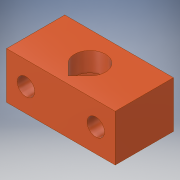
# Autodesk Inventor part: X-axis Holder coupler
Saved by Autodesk Inventor 2018 (Build 220112000, 112)
## iProperties
Created: 2013-10-26
Part Number: X-axis Holder coupler
Material: ABS Plastic
Document SubType Name: Modeling
Designer: Gabriel Smolnycki
Mass: 4.42597 g
Surface Area: 24.3848 cm^2
Volume: 4.17544 cm^3
Density: 1.06 g/cm^3
Appearance: Smooth - Light Orange
Author: Gabriel Smolnycki
Sending System: SolidWorks 2017
Last Author: Gabriel Smolnycki
Last Saved: 2017-09-14
Autodesk Inventor part; units mm, degrees
ref_plane "YZ Plane" through (0, 0, 0) normal (1, 0, 0) x (0, 1, 0)
ref_plane "XZ Plane" through (0, 0, 0) normal (0, 1, 0) x (-1, 0, 0)
ref_plane "XY Plane" through (0, 0, 0) normal (0, 0, 1) x (1, 0, 0)
sketch "Sketch1" plane through (0, 0, 0) normal (0, 0, 1) x (1, 0, 0)
  line L0 (-14, 0) -> (-14, 12)
  line L1 (14, 0) -> (14, 12)
  line L2 (14, 0) -> (-14, 0)
  line L3 (14, 12) -> (-14, 12)
  constraints: 8 end point, 2 horizontal, 2 vertical
extrude "Extrusion3" add sketch "Sketch1" against normal blind 15 draft 0
sketch "Sketch2" plane through (-14, 12, 0) normal (0, 1, 0) x (1, 0, 0)
  arc A0 (16.8284, 4.6716) -> (11.1716, 4.6716) centre (14, 7.5) ccw
  line L0 (11.1716, 4.6716) -> (14, 1.8431)
  line L1 (14, 1.8431) -> (16.8284, 4.6716)
  constraints: 4 end point, 2 perpendicular, 2 point on circle, 1 centre point
extrude "Extrusion2" cut sketch "Sketch2" against normal blind 5
sketch "Sketch3" plane through (-14, 7, 0) normal (0, 1, 0) x (1, 0, 0)
  arc A0 (15.591, 5.909) -> (12.409, 5.909) centre (14, 7.5) ccw
  line L0 (12.409, 5.909) -> (14, 4.318)
  line L1 (14, 4.318) -> (15.591, 5.909)
  constraints: 4 end point, 2 perpendicular, 2 point on circle, 1 centre point
extrude "Extrusion1" cut sketch "Sketch3" against normal blind 7
hole "Hole2" at (9, 6, 0) direction (0, 0, -1) diameter 4.5 depth 15
sketch "Sketch4" plane through (0, 0, 0) normal (0, 0, 1) x (1, 0, 0)
  point P0 (9, 6)
hole "Hole1" at (-9, 6, 0) direction (0, 0, -1) diameter 4.5 depth 15
sketch "Sketch5" plane through (0, 0, 0) normal (0, 0, 1) x (1, 0, 0)
  point P0 (-9, 6)
body "Solid3"
